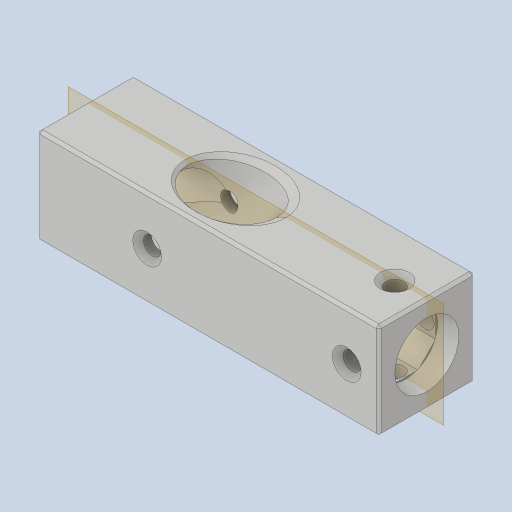
# Autodesk Inventor part: holderHolder
Saved by Autodesk Inventor 2024 (Build 280153000, 153)
## iProperties
Created: 2019-08-19
Part Number: holderHolder
Material: Generic
Document SubType Name: Modeling
Designer: Daniel
Density: 1 g/cm^3
Appearance: Default
Author: Daniel
Autodesk Inventor part; units mm, degrees
ref_plane "YZ Plane" through (0, 0, 0) normal (1, 0, 0) x (0, 1, 0)
ref_plane "XZ Plane" through (0, 0, 0) normal (0, 1, 0) x (-1, 0, 0)
ref_plane "XY Plane" through (0, 0, 0) normal (0, 0, 1) x (1, 0, 0)
sketch "Sketch1" plane through (0, 0, 0) normal (0, 1, 0) x (-1, 0, 0)
  line L0 (0, 0) -> (-60, 0)
  line L1 (-60, 0) -> (-60, -18)
  line L2 (-60, -18) -> (0, -18)
  line L3 (0, -18) -> (0, 0)
  dimension "d0" = 60
  dimension "d1" = 18
  constraints: 8 end point, 2 parallel, 1 horizontal, 1 perpendicular
  measures "d0" distance of L1.end L2.end
  measures "d1" distance of L2.end L0.start
extrude "Extrusion1" add sketch "Sketch1" along normal blind 18
sketch "Sketch2" plane through (60, 0, 0) normal (1, 0, 0) x (0, 0, -1)
  line L0 (14.7, 6.639) -> (11.361, 3.3)
  line L1 (11.361, 3.3) -> (6.639, 3.3)
  line L2 (6.639, 3.3) -> (3.3, 6.639)
  line L3 (3.3, 6.639) -> (3.3, 11.361)
  line L4 (3.3, 11.361) -> (6.639, 14.7)
  line L5 (6.639, 14.7) -> (11.361, 14.7)
  line L6 (11.361, 14.7) -> (14.7, 11.361)
  line L7 (14.7, 11.361) -> (14.7, 6.639)
  line L8 (0, 18) -> (18, 18) construction
  line L9 (9, 18) -> (9, 0) construction
  line L10 (0, 0) -> (18, 0) construction
  line L11 (0, 0) -> (0, 18) construction
  line L12 (0, 9) -> (18, 9) construction
  line L13 (18, 0) -> (18, 18) construction
  point P0 (9, 9)
  dimension "d4" = 11.4
  dimension "d28" = 0
  constraints: 20 end point, 5 midpoint, 17 other
  measures "d4" distance between parallel lines of L1 L5
  measures "d28" angle of L12 L5
extrude "Extrusion2" cut sketch "Sketch2" against normal blind 18
sketch "Sketch3" plane through (42, 0, 0) normal (1, 0, 0) x (0, 0, -1)
  line L0 (14.7, 6.639) -> (11.361, 3.3) projected
  line L1 (14.7, 11.361) -> (14.7, 6.639) projected
  line L2 (11.361, 14.7) -> (14.7, 11.361) projected
  line L3 (6.639, 14.7) -> (11.361, 14.7) projected
  line L4 (3.3, 11.361) -> (6.639, 14.7) projected
  line L5 (3.3, 6.639) -> (3.3, 11.361) projected
  line L6 (6.639, 3.3) -> (3.3, 6.639) projected
  line L7 (11.361, 3.3) -> (6.639, 3.3) projected
  circle A0 centre (9, 9) radius 4
  point P0 (0, 0)
  dimension "d7" = 8
  constraints: 1 centre point
  measures "d7" diameter of A0
extrude "Extrusion3" cut sketch "Sketch3" against normal through all contours A0
sketch "Sketch4" plane through (0, 0, -18) normal (-1, 0, 0) x (0, 0, 1)
  circle A0 centre (9, 9) radius 4 projected
  circle A1 centre (9, 9) radius 6.5
  point P0 (18, 0)
  dimension "d10" = 13
  constraints: 1 centre point, 1 coincident
  measures "d10" diameter of A1
extrude "Extrusion4" cut sketch "Sketch4" against normal blind 20
ref_plane "Work Plane1" through (0, 0, -18) normal (-0.6427876, -0.7660444, 0) x (0, 0, 1)
sketch "Sketch5" plane through (-4.716, 3.9572, 0) normal (0.6427876, 0.7660444, 0) x (0.7660444, -0.6427876, 0)
  circle A0 centre (16.1564, 9) radius 6.45
  line L0 (6.1564, 18) -> (6.1564, 0) construction
  line L1 (6.1564, 9) -> (16.1564, 9) construction
  dimension "d13" = 12.9
  dimension "d27" = 10
  constraints: 2 end point, 1 centre point, 1 horizontal, 1 midpoint
  measures "d13" diameter of A0
  measures "d27" distance from line of L0 L1.end
extrude "Extrusion5" cut sketch "Sketch5" along normal through all
ref_plane "Work Plane3" through (0, 0, -18) normal (-0.5, -0.8660254, 0) x (0, 0, 1)
ref_plane "Work Plane2" through (42, -7.45, -11.361) normal (0, 1, 0) x (1, 0, 0)
sketch "Sketch9" plane through (60, 0, 0) normal (1, 0, 0) x (0, 0, -1)
  arc A0 (2.761, 10.8234) -> (15.239, 10.8234) centre (9, 9) ccw projected
  circle A1 centre (9, 9) radius 6
  line L0 (0, 0) -> (0, 18) projected
  line L1 (0, 18) -> (18, 18) projected
  line L2 (0, 0) -> (18, 0) projected
  line L3 (18, 0) -> (18, 18) projected
  dimension "d49" = 12
  constraints: 1 centre point, 1 coincident
  measures "d49" diameter of A1
extrude "Extrusion9" add sketch "Sketch9" along normal blind 4
sketch "Sketch6" plane through (0, 0, 0) normal (0, 0, 1) x (1, 0, 0)
  line L0 (0, 0) -> (0, 18) construction
  line L1 (0, 9) -> (50.6885, 9) construction
  circle A0 centre (20.606, 9) radius 1.7
  line L2 (21.4739, 0) -> (4.6342, 0) projected
  line L3 (19.738, 18) -> (36.5777, 18) projected
  line L4 (19.738, 18) -> (21.4739, 0) construction
  line L5 (36.5777, 18) -> (4.6342, 0) construction
  dimension "d23" = 3.4
  constraints: 6 end point, 2 midpoint, 1 centre point, 1 point on line
  measures "d23" diameter of A0
extrude "Extrusion6" cut sketch "Sketch6" against normal through all
sketch "Sketch10" plane through (0, 0, -18) normal (-0.5, -0.8660254, 0) x (0, 0, 1)
  circle A0 centre (9, -13.3453) radius 6.45
  line L0 (0, 0) -> (18, 0) projected
  line L1 (18, -11.6453) -> (18, -15.0453) projected
  point P0 (9, 0)
  point P1 (9, 0)
  point P2 (18, -13.3453)
  dimension "d59" = 12.9
  constraints: 3 midpoint, 2 vertical alignment, 1 centre point, 1 horizontal alignment
  measures "d59" diameter of A0
extrude "Extrusion10" [suppressed]
sketch "Sketch7" plane through (42, -7.45, -11.361) normal (0, 1, 0) x (1, 0, 0)
  circle A0 centre (16, -2.361) radius 1.7
  line L0 (18, -0.4875) -> (18, -4.2345) projected
  line L1 (18, 0) -> (0, 0) projected
  line L2 (0, 0) -> (0, -4.722) projected
  line L3 (18, -4.722) -> (0, -4.722) projected
  line L4 (18, 0) -> (18, -0.4875) projected
  line L5 (18, -4.2345) -> (18, -4.722) projected
  point P0 (-42, -11.361)
  dimension "d30" = 3.4
  dimension "d31" = 2.361
  dimension "d32" = 2.361
  dimension "d33" = 2
  constraints: 1 centre point
  measures "d30" diameter of A0
  measures "d31" distance from line of L1 A0.centre
  measures "d32" distance from line of L3 A0.centre
  measures "d33" distance from line of L0 A0.centre
extrude "Extrusion7" cut sketch "Sketch7" along normal through all contours A0
pattern_circular "Circular Pattern1" count 4 over 360 about axis through (60, 9, -9) along (1, 0, 0) of "Extrusion7"
ref_plane "Work Plane4" through (0, 0, -9) normal (0, 0, 1) x (1, 0, 0)
sketch "Sketch8" plane through (0, 0, 0) normal (0, -1, 0) x (1, 0, 0)
  line L0 (32, -18) -> (46, -18) construction
  line L1 (46, -18) -> (46, 0) construction
  line L2 (46, 0) -> (32, 0) construction
  line L3 (32, 0) -> (32, -18) construction
  line L4 (0, 0) -> (64, 0) projected
  line L5 (0, 0) -> (64, 0) projected
  line L6 (0, -18) -> (64, -18) projected
  circle A0 centre (58, -9) radius 1.7 projected
  spline S0 degree 2 poles (35.027, -5.8844) (35.027, -6.082) (34.8862, -6.4377) (34.7602, -6.5612) knots 0 0 0 1 2 2 2
  spline S1 degree 2 poles (34.7602, -6.5612) (34.6021, -6.7168) (34.1748, -6.8773) (33.8488, -6.8773) knots 0 0 0 1 2 2 2
  line L7 (33.8488, -6.8773) -> (33.5054, -6.8773)
  line L8 (33.5054, -6.8773) -> (33.5054, -8.0135)
  line L9 (33.5054, -8.0135) -> (33.1004, -8.0135)
  line L10 (33.1004, -8.0135) -> (33.1004, -4.9655)
  line L11 (33.1004, -4.9655) -> (33.8661, -4.9655)
  spline S2 degree 2 poles (33.8661, -4.9655) (34.1378, -4.9655) (34.5182, -5.0545) (34.6639, -5.1557) knots 0 0 0 1 2 2 2
  spline S3 degree 2 poles (34.6639, -5.1557) (34.8343, -5.2718) (35.027, -5.63) (35.027, -5.8844) knots 0 0 0 1 2 2 2
  spline S4 degree 2 poles (34.6046, -5.8967) (34.6046, -5.7387) (34.4959, -5.5065) (34.3848, -5.4324) knots 0 0 0 1 2 2 2
  spline S5 degree 2 poles (34.3848, -5.4324) (34.2884, -5.3682) (34.0316, -5.3163) (33.8414, -5.3163) knots 0 0 0 1 2 2 2
  line L12 (33.8414, -5.3163) -> (33.5054, -5.3163)
  line L13 (33.5054, -5.3163) -> (33.5054, -6.5315)
  line L14 (33.5054, -6.5315) -> (33.7821, -6.5315)
  spline S6 degree 2 poles (33.7821, -6.5315) (34.0291, -6.5315) (34.3329, -6.4525) (34.4317, -6.3487) knots 0 0 0 1 2 2 2
  spline S7 degree 2 poles (34.4317, -6.3487) (34.5231, -6.2574) (34.6046, -6.0425) (34.6046, -5.8967) knots 0 0 0 1 2 2 2
  line L15 (37.287, -6.9663) -> (36.924, -6.9663)
  line L16 (36.924, -6.9663) -> (36.924, -8.0135)
  line L17 (36.924, -8.0135) -> (36.5312, -8.0135)
  line L18 (36.5312, -8.0135) -> (36.5312, -6.9663)
  line L19 (36.5312, -6.9663) -> (35.1851, -6.9663)
  line L20 (35.1851, -6.9663) -> (35.1851, -6.5365)
  line L21 (35.1851, -6.5365) -> (36.5485, -4.9655)
  line L22 (36.5485, -4.9655) -> (36.924, -4.9655)
  line L23 (36.924, -4.9655) -> (36.924, -6.6377)
  line L24 (36.924, -6.6377) -> (37.287, -6.6377)
  line L25 (37.287, -6.6377) -> (37.287, -6.9663)
  line L26 (36.5312, -6.6377) -> (36.5312, -5.4472)
  line L27 (36.5312, -5.4472) -> (35.5062, -6.6377)
  line L28 (35.5062, -6.6377) -> (36.5312, -6.6377)
  spline S8 degree 2 poles (39.5101, -6.4895) (39.5101, -7.3096) (39.0333, -8.0778) (38.5369, -8.0778) knots 0 0 0 1 2 2 2
  spline S9 degree 2 poles (38.5369, -8.0778) (38.033, -8.0778) (37.5612, -7.2948) (37.5612, -6.492) knots 0 0 0 1 2 2 2
  spline S10 degree 2 poles (37.5612, -6.492) (37.5612, -5.667) (38.0379, -4.9038) (38.5369, -4.9038) knots 0 0 0 1 2 2 2
  spline S11 degree 2 poles (38.5369, -4.9038) (39.0383, -4.9038) (39.5101, -5.6942) (39.5101, -6.4895) knots 0 0 0 1 2 2 2
  spline S12 degree 2 poles (38.9864, -7.4183) (39.0457, -7.2676) (39.0951, -6.8032) (39.0951, -6.4895) knots 0 0 0 1 2 2 2
  spline S13 degree 2 poles (39.0951, -6.4895) (39.0951, -6.1758) (39.0457, -5.714) (38.9839, -5.5583) knots 0 0 0 1 2 2 2
  spline S14 degree 2 poles (38.9839, -5.5583) (38.9222, -5.4027) (38.7073, -5.2422) (38.5369, -5.2422) knots 0 0 0 1 2 2 2
  spline S15 degree 2 poles (38.5369, -5.2422) (38.3664, -5.2422) (38.1466, -5.4027) (38.0824, -5.5633) knots 0 0 0 1 2 2 2
  spline S16 degree 2 poles (38.0824, -5.5633) (38.0206, -5.7189) (37.9762, -6.1931) (37.9762, -6.492) knots 0 0 0 1 2 2 2
  spline S17 degree 2 poles (37.9762, -6.492) (37.9762, -6.8131) (38.0157, -7.2429) (38.0799, -7.4109) knots 0 0 0 1 2 2 2
  spline S18 degree 2 poles (38.0799, -7.4109) (38.1392, -7.5689) (38.359, -7.7394) (38.5369, -7.7394) knots 0 0 0 1 2 2 2
  spline S19 degree 2 poles (38.5369, -7.7394) (38.7048, -7.7394) (38.9247, -7.5788) (38.9864, -7.4183) knots 0 0 0 1 2 2 2
  line L29 (40.5549, -8.0135) -> (40.0658, -8.0135)
  line L30 (40.0658, -8.0135) -> (40.0658, -7.4306)
  line L31 (40.0658, -7.4306) -> (40.5549, -7.4306)
  line L32 (40.5549, -7.4306) -> (40.5549, -8.0135)
  spline S20 degree 2 poles (43.0669, -6.4895) (43.0669, -7.3096) (42.5902, -8.0778) (42.0937, -8.0778) knots 0 0 0 1 2 2 2
  spline S21 degree 2 poles (42.0937, -8.0778) (41.5898, -8.0778) (41.118, -7.2948) (41.118, -6.492) knots 0 0 0 1 2 2 2
  spline S22 degree 2 poles (41.118, -6.492) (41.118, -5.667) (41.5948, -4.9038) (42.0937, -4.9038) knots 0 0 0 1 2 2 2
  spline S23 degree 2 poles (42.0937, -4.9038) (42.5951, -4.9038) (43.0669, -5.6942) (43.0669, -6.4895) knots 0 0 0 1 2 2 2
  spline S24 degree 2 poles (42.5432, -7.4183) (42.6025, -7.2676) (42.6519, -6.8032) (42.6519, -6.4895) knots 0 0 0 1 2 2 2
  spline S25 degree 2 poles (42.6519, -6.4895) (42.6519, -6.1758) (42.6025, -5.714) (42.5408, -5.5583) knots 0 0 0 1 2 2 2
  spline S26 degree 2 poles (42.5408, -5.5583) (42.479, -5.4027) (42.2641, -5.2422) (42.0937, -5.2422) knots 0 0 0 1 2 2 2
  spline S27 degree 2 poles (42.0937, -5.2422) (41.9233, -5.2422) (41.7034, -5.4027) (41.6392, -5.5633) knots 0 0 0 1 2 2 2
  spline S28 degree 2 poles (41.6392, -5.5633) (41.5775, -5.7189) (41.533, -6.1931) (41.533, -6.492) knots 0 0 0 1 2 2 2
  spline S29 degree 2 poles (41.533, -6.492) (41.533, -6.8131) (41.5725, -7.2429) (41.6367, -7.4109) knots 0 0 0 1 2 2 2
  spline S30 degree 2 poles (41.6367, -7.4109) (41.696, -7.5689) (41.9159, -7.7394) (42.0937, -7.7394) knots 0 0 0 1 2 2 2
  spline S31 degree 2 poles (42.0937, -7.7394) (42.2617, -7.7394) (42.4815, -7.5788) (42.5432, -7.4183) knots 0 0 0 1 2 2 2
  spline S32 degree 2 poles (45.0009, -5.6917) (45.0009, -6.0202) (44.5514, -6.4698) (44.2228, -6.4698) knots 0 0 0 1 2 2 2
  spline S33 degree 2 poles (44.2228, -6.4698) (43.8968, -6.4698) (43.4423, -6.0227) (43.4423, -5.6917) knots 0 0 0 1 2 2 2
  spline S34 degree 2 poles (43.4423, -5.6917) (43.4423, -5.3632) (43.8919, -4.9137) (44.2228, -4.9137) knots 0 0 0 1 2 2 2
  spline S35 degree 2 poles (44.2228, -4.9137) (44.5514, -4.9137) (45.0009, -5.3632) (45.0009, -5.6917) knots 0 0 0 1 2 2 2
  spline S36 degree 2 poles (44.6798, -5.6917) (44.6798, -5.4941) (44.418, -5.2249) (44.2228, -5.2249) knots 0 0 0 1 2 2 2
  spline S37 degree 2 poles (44.2228, -5.2249) (44.0252, -5.2249) (43.7634, -5.4941) (43.7634, -5.6917) knots 0 0 0 1 2 2 2
  spline S38 degree 2 poles (43.7634, -5.6917) (43.7634, -5.8918) (44.0302, -6.1586) (44.2228, -6.1586) knots 0 0 0 1 2 2 2
  spline S39 degree 2 poles (44.2228, -6.1586) (44.418, -6.1586) (44.6798, -5.8869) (44.6798, -5.6917) knots 0 0 0 1 2 2 2
  line L33 (36.4584, -13.032) -> (35.9322, -13.032)
  line L34 (35.9322, -13.032) -> (34.9689, -11.8192)
  line L35 (34.9689, -11.8192) -> (34.5046, -11.8192)
  line L36 (34.5046, -11.8192) -> (34.5046, -13.032)
  line L37 (34.5046, -13.032) -> (34.0995, -13.032)
  line L38 (34.0995, -13.032) -> (34.0995, -9.984)
  line L39 (34.0995, -9.984) -> (34.885, -9.984)
  spline S40 degree 2 poles (34.885, -9.984) (35.1468, -9.984) (35.5, -10.0408) (35.6605, -10.1445) knots 0 0 0 1 2 2 2
  spline S41 degree 2 poles (35.6605, -10.1445) (35.8211, -10.2483) (36.0063, -10.5719) (36.0063, -10.8114) knots 0 0 0 1 2 2 2
  spline S42 degree 2 poles (36.0063, -10.8114) (36.0063, -11.1449) (35.6655, -11.5969) (35.374, -11.7056) knots 0 0 0 1 2 2 2
  line L40 (35.374, -11.7056) -> (36.4584, -13.032)
  spline S43 degree 2 poles (35.584, -10.8436) (35.584, -10.7102) (35.4901, -10.5052) (35.3913, -10.4385) knots 0 0 0 1 2 2 2
  spline S44 degree 2 poles (35.3913, -10.4385) (35.3049, -10.3817) (35.0751, -10.3347) (34.9072, -10.3347) knots 0 0 0 1 2 2 2
  line L41 (34.9072, -10.3347) -> (34.5046, -10.3347)
  line L42 (34.5046, -10.3347) -> (34.5046, -11.4808)
  line L43 (34.5046, -11.4808) -> (34.8603, -11.4808)
  spline S45 degree 2 poles (34.8603, -11.4808) (35.0356, -11.4808) (35.3147, -11.4191) (35.4111, -11.3227) knots 0 0 0 1 2 2 2
  spline S46 degree 2 poles (35.4111, -11.3227) (35.5, -11.2388) (35.584, -11.0016) (35.584, -10.8436) knots 0 0 0 1 2 2 2
  spline S47 degree 2 poles (38.5109, -11.508) (38.5109, -12.328) (38.0342, -13.0962) (37.5378, -13.0962) knots 0 0 0 1 2 2 2
  spline S48 degree 2 poles (37.5378, -13.0962) (37.0339, -13.0962) (36.5621, -12.3132) (36.5621, -11.5105) knots 0 0 0 1 2 2 2
  spline S49 degree 2 poles (36.5621, -11.5105) (36.5621, -10.6855) (37.0388, -9.9222) (37.5378, -9.9222) knots 0 0 0 1 2 2 2
  spline S50 degree 2 poles (37.5378, -9.9222) (38.0392, -9.9222) (38.5109, -10.7126) (38.5109, -11.508) knots 0 0 0 1 2 2 2
  spline S51 degree 2 poles (37.9873, -12.4367) (38.0466, -12.286) (38.096, -11.8217) (38.096, -11.508) knots 0 0 0 1 2 2 2
  spline S52 degree 2 poles (38.096, -11.508) (38.096, -11.1943) (38.0466, -10.7324) (37.9848, -10.5768) knots 0 0 0 1 2 2 2
  spline S53 degree 2 poles (37.9848, -10.5768) (37.9231, -10.4212) (37.7082, -10.2606) (37.5378, -10.2606) knots 0 0 0 1 2 2 2
  spline S54 degree 2 poles (37.5378, -10.2606) (37.3673, -10.2606) (37.1475, -10.4212) (37.0833, -10.5817) knots 0 0 0 1 2 2 2
  spline S55 degree 2 poles (37.0833, -10.5817) (37.0215, -10.7373) (36.9771, -11.2116) (36.9771, -11.5105) knots 0 0 0 1 2 2 2
  spline S56 degree 2 poles (36.9771, -11.5105) (36.9771, -11.8316) (37.0166, -12.2613) (37.0808, -12.4293) knots 0 0 0 1 2 2 2
  spline S57 degree 2 poles (37.0808, -12.4293) (37.1401, -12.5874) (37.3599, -12.7578) (37.5378, -12.7578) knots 0 0 0 1 2 2 2
  spline S58 degree 2 poles (37.5378, -12.7578) (37.7057, -12.7578) (37.9255, -12.5973) (37.9873, -12.4367) knots 0 0 0 1 2 2 2
  line L44 (39.5558, -13.032) -> (39.0667, -13.032)
  line L45 (39.0667, -13.032) -> (39.0667, -12.4491)
  line L46 (39.0667, -12.4491) -> (39.5558, -12.4491)
  line L47 (39.5558, -12.4491) -> (39.5558, -13.032)
  spline S59 degree 2 poles (42.0678, -11.508) (42.0678, -12.328) (41.591, -13.0962) (41.0946, -13.0962) knots 0 0 0 1 2 2 2
  spline S60 degree 2 poles (41.0946, -13.0962) (40.5907, -13.0962) (40.1189, -12.3132) (40.1189, -11.5105) knots 0 0 0 1 2 2 2
  spline S61 degree 2 poles (40.1189, -11.5105) (40.1189, -10.6855) (40.5956, -9.9222) (41.0946, -9.9222) knots 0 0 0 1 2 2 2
  spline S62 degree 2 poles (41.0946, -9.9222) (41.596, -9.9222) (42.0678, -10.7126) (42.0678, -11.508) knots 0 0 0 1 2 2 2
  spline S63 degree 2 poles (41.5441, -12.4367) (41.6034, -12.286) (41.6528, -11.8217) (41.6528, -11.508) knots 0 0 0 1 2 2 2
  spline S64 degree 2 poles (41.6528, -11.508) (41.6528, -11.1943) (41.6034, -10.7324) (41.5416, -10.5768) knots 0 0 0 1 2 2 2
  spline S65 degree 2 poles (41.5416, -10.5768) (41.4799, -10.4212) (41.265, -10.2606) (41.0946, -10.2606) knots 0 0 0 1 2 2 2
  spline S66 degree 2 poles (41.0946, -10.2606) (40.9241, -10.2606) (40.7043, -10.4212) (40.6401, -10.5817) knots 0 0 0 1 2 2 2
  spline S67 degree 2 poles (40.6401, -10.5817) (40.5783, -10.7373) (40.5339, -11.2116) (40.5339, -11.5105) knots 0 0 0 1 2 2 2
  spline S68 degree 2 poles (40.5339, -11.5105) (40.5339, -11.8316) (40.5734, -12.2613) (40.6376, -12.4293) knots 0 0 0 1 2 2 2
  spline S69 degree 2 poles (40.6376, -12.4293) (40.6969, -12.5874) (40.9167, -12.7578) (41.0946, -12.7578) knots 0 0 0 1 2 2 2
  spline S70 degree 2 poles (41.0946, -12.7578) (41.2625, -12.7578) (41.4824, -12.5973) (41.5441, -12.4367) knots 0 0 0 1 2 2 2
  spline S71 degree 2 poles (44.0018, -10.7102) (44.0018, -11.0387) (43.5522, -11.4882) (43.2237, -11.4882) knots 0 0 0 1 2 2 2
  spline S72 degree 2 poles (43.2237, -11.4882) (42.8977, -11.4882) (42.4432, -11.0412) (42.4432, -10.7102) knots 0 0 0 1 2 2 2
  spline S73 degree 2 poles (42.4432, -10.7102) (42.4432, -10.3817) (42.8927, -9.9321) (43.2237, -9.9321) knots 0 0 0 1 2 2 2
  spline S74 degree 2 poles (43.2237, -9.9321) (43.5522, -9.9321) (44.0018, -10.3817) (44.0018, -10.7102) knots 0 0 0 1 2 2 2
  spline S75 degree 2 poles (43.6807, -10.7102) (43.6807, -10.5126) (43.4189, -10.2433) (43.2237, -10.2433) knots 0 0 0 1 2 2 2
  spline S76 degree 2 poles (43.2237, -10.2433) (43.0261, -10.2433) (42.7643, -10.5126) (42.7643, -10.7102) knots 0 0 0 1 2 2 2
  spline S77 degree 2 poles (42.7643, -10.7102) (42.7643, -10.9102) (43.0311, -11.177) (43.2237, -11.177) knots 0 0 0 1 2 2 2
  spline S78 degree 2 poles (43.2237, -11.177) (43.4189, -11.177) (43.6807, -10.9053) (43.6807, -10.7102) knots 0 0 0 1 2 2 2
  point P0 (60, 0)
  dimension "roll" = 0
  dimension "pitch" = 40
  dimension "d53" = 14
  dimension "d68" = 12
  constraints: 2 collinear, 2 other
  measures "d53" distance between parallel lines of L1 L3
  measures "d68" distance from line of A0.centre L1
extrude "Extrusion8" cut sketch "Sketch8" against normal blind 0.75 contours S0 S1 L7 L8 L9 L10 L11 S2 S3 | L15 L16 L17 L18 L19 L20 L21 L22 L23 L24 L25 | S8 S9 S10 S11 | L29 L30 L31 L32 | S20 S21 S22 S23 | S32 S33 S34 S35 | L33 L34 L35 L36 L37 L38 L39 S40 S41 S42 L40 | S47 S48 S49 S50 | L44 L45 L46 L47 | S59 S60 S61 S62 | S71 S72 S73 S74
sketch "Sketch11" plane through (64, 0, 0) normal (1, 0, 0) x (0, 0, -1)
  line L0 (18, 0) -> (0, 0) projected
  line L1 (18, 0) -> (23.25, 0)
  line L2 (23.25, 0) -> (23.25, 2)
  line L3 (23.25, 2) -> (18, 2)
  line L4 (18, 2) -> (18, 0)
  line L5 (23.25, 2) -> (21.25, 2)
  line L6 (21.25, 2) -> (21.25, 8)
  line L7 (21.25, 8) -> (23.25, 8)
  line L8 (23.25, 8) -> (23.25, 2)
  line L9 (18, 0) -> (18, 18) projected
  line L10 (18, 18) -> (0, 18) projected
  dimension "d63" = 3.25
  dimension "d64" = 2
  dimension "d65" = 2
  dimension "d69" = 6
  constraints: 16 end point, 4 parallel, 2 horizontal, 2 perpendicular
  measures "d63" distance between parallel lines of L6 L9
  measures "d64" distance of L1.end L2.end
  measures "d65" distance of L6.end L7.end
  measures "d69" distance between parallel lines of L3 L7
extrude "Extrusion11" [suppressed]
sketch "Sketch13" plane through (64, 0, -23.25) normal (0, 0, -1) x (-1, 0, 0)
  circle A0 centre (6, 9) radius 1.7 construction
  circle A1 centre (43.394, 9) radius 1.7 construction
  circle A2 centre (6, 9) radius 4
  circle A3 centre (43.394, 9) radius 1.7 projected
  circle A4 centre (43.394, 9) radius 4
  point P0 (64, 0)
  dimension "d70" = 8
  constraints: 2 centre point, 2 coincident, 1 equal radius
  measures "d70" diameter of A2
extrude "Extrusion12" [suppressed]
mirror "Mirror1" [suppressed]
chamfer "Chamfer2" distance 0.5 angle 45 9 edges at (32, 18, 0) (32, 18, -18) (0, 9, -18) (0, 0, -9) (0, 9, 0) (0, 18, -9) (64, 18, -9) (64, 9, 0) (64, 9, -18)
chamfer "Chamfer3" distance 1 angle 45 9 edges at (18.906, 9, 0) (18.906, 9, -18) (56.3, 0, -9) (56.3, 18, -9) (0, 9, -15.5) (19.738, 18, -9) (4.6342, 0, -9) (56.3, 9, 0) (56.3, 9, -18)
chamfer "Chamfer4" distance 0.5 angle 45 3 edges at (32, 0, 0) (32, 0, -18) (64, 0, -9)
equation "\"d31\" = d32"
equation "\"roll\" = 0"
equation "\"pitch\" = 40deg"
equation "\"d25\" = -pitch"
equation "\"d58\" = -pitch2"
equation "\"pitch2\" = 30deg"
body "Solid1"
